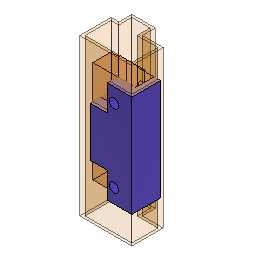
design (Autodesk Fusion 360 design; units mm, degrees)
Autodesk Fusion 360 part; units mm, degrees
note: some values were not read from the file. Chosen so that the rebuilt part matches the saved one: which bodies a step acts on.
sketch "Sketch1" plane through (0, 0, 0) normal (0, 0, 1) x (1, 0, 0) in component "铝槽"
  line L0 (0, 0) -> (18, 0)
  line L1 (18, 0) -> (18, 10)
  line L2 (18, 10) -> (10, 10)
  line L3 (10, 10) -> (10, 15)
  line L4 (10, 15) -> (3, 15)
  line L5 (3, 15) -> (3, 10)
  line L6 (3, 10) -> (0, 10)
  line L7 (0, 10) -> (0, 0)
  line L8 (-1, -1) -> (19, -1)
  line L9 (19, -1) -> (19, 11)
  line L10 (19, 11) -> (11, 11)
  line L11 (11, 11) -> (11, 16)
  line L12 (11, 16) -> (2, 16)
  line L13 (2, 16) -> (2, 11)
  line L14 (2, 11) -> (-1, 11)
  line L15 (-1, 11) -> (-1, -1)
  dimension "d1" = 18
  dimension "d2" = 10
  dimension "d3" = 8
  dimension "d4" = 5
  dimension "d5" = 7
  dimension "d6" = 1
  constraint coincident L0.start L7.end
  constraint horizontal L0
  constraint perpendicular L0 L1
  constraint perpendicular L1 L2
  constraint perpendicular L2 L3
  constraint perpendicular L3 L4
  constraint perpendicular L4 L5
  constraint perpendicular L5 L6
  constraint perpendicular L0 L7
  constraint equal L3 L5
  measures "d1" distance of L0.start L0.end
  measures "d2" distance of L0.end L1.end
  measures "d3" distance of L1.end L2.end
  measures "d4" distance of L2.end L3.end
  measures "d5" distance of L3.end L4.end
extrude "Extrude1" add sketch "Sketch1" along normal blind 60 makes body 1 in component "铝槽"
sketch "Sketch1 (2)" plane through (0, 0, 0) normal (0, 1, 0) x (1, 0, 0) in component "门铰"
  line L0 (0, -19.5) -> (0, 19.5)
  line L1 (-16, -9.5) -> (-16, 9.5)
  line L2 (0, -19.5) -> (-9.5, -19.5)
  line L3 (0, 19.5) -> (-9.5, 19.5)
  line L4 (-16, -9.5) -> (-9.5, -9.5)
  line L5 (-9.5, -9.5) -> (-9.5, -19.5)
  line L6 (-16, 9.5) -> (-9.5, 9.5)
  line L7 (-9.5, 9.5) -> (-9.5, 19.5)
  line L8 (0, 0) -> (-16, 0) construction
  circle A0 centre (-6.9, -14) radius 1.75
  circle A1 centre (-6.9, 14) radius 1.75
  dimension "d9" = 39
  dimension "d10" = 19
  dimension "d11" = 9.5
  dimension "d12" = 16
  dimension "d14" = 3.5
  dimension "d15" = 6.9
  dimension "d16" = 28
  constraint vertical L0
  constraint midpoint L8.start L0
  constraint vertical L1
  constraint perpendicular L0 L2
  constraint perpendicular L0 L3
  constraint equal L2 L3
  constraint perpendicular L1 L4
  constraint vertical L5
  constraint perpendicular L1 L6
  constraint vertical L7
  constraint equal L5 L7
  constraint coincident L8.start origin
  constraint midpoint L1 L8.end
  constraint symmetric L8 A0 A1
  measures "d9" distance of L0.start L0.end
  measures "d10" distance of L1.start L1.end
  measures "d11" distance of L0.start L2.end
  measures "d12" distance of L0 L1
  measures "d14" diameter of A0
  measures "d15" distance of L0 A0.centre
  measures "d16" distance of A0.centre A1.centre
extrude "Extrude1'" add sketch "Sketch1 (2)" along normal blind 11 separate body makes body 2 in component "门铰"
ref_plane "WorkPlane1" through (0, 5.5, 0) normal (1, 0, 0) x (0, 0, -1) in component "门铰"
sketch "Sketch2" plane through (0, 5.5, 0) normal (1, 0, 0) x (0, 1, 0) in component "门铰"
  line L0 (-5.5, 9.5) -> (-1.5, 9.5)
  line L1 (-5.5, -9.5) -> (-1.5, -9.5)
  line L2 (-5.5, 19.5) -> (-5.5, -19.5)
  line L3 (-5.5, -19.5) -> (5.5, -19.5)
  line L4 (5.5, -19.5) -> (5.5, 19.5)
  line L5 (5.5, 19.5) -> (-5.5, 19.5)
  line L6 (-1.5, 9.5) -> (-1.5, 19.5)
  line L7 (-1.5, -9.5) -> (-1.5, -19.5)
  line L8 (-1.5, 9.5) -> (5.5, 9.5)
  line L9 (-1.5, -9.5) -> (5.5, -9.5)
  point P0 (-5.5, 9.5)
  point P1 (-5.5, -9.5)
  dimension "d20" = 4
  constraint coincident P0 L0.start
  constraint horizontal L0
  constraint coincident P1 L1.start
  constraint horizontal L1
  constraint equal L0 L1
  constraint coincident L5 L6.end
  constraint perpendicular L5 L6
  constraint coincident L3 L7.end
  constraint perpendicular L3 L7
  constraint coincident L4 L8.end
  constraint perpendicular L4 L8
  constraint coincident L4 L9.end
  constraint perpendicular L4 L9
  measures "d20" distance of P0 L0.end
extrude "Extrude2" cut sketch "Sketch2" against normal up to surface (7 mm away) from surface at -2.5 contours L4 L5 L6 L8 | L3 L4 L7 L9 bodies 2 in component "门铰"
combine "Combine1" operation cut target body 1 tool bodies 2 body 2 seen with x (1, 0, 0) y (0, 1, 0) z (0, 0, 1) at (19, -1, 30) keep tools makes body 3 at (13.8413, -0.6667, 44.1742) makes body 4 at (13.8413, -0.6667, 16.1742) in component "铝槽"
sketch "Sketch1 (3)" plane through (0, 11.9627, 0) normal (0, 1, 0) x (-1, 0, 0) in component "填块"
  line L0 (-12.0433, -6.2222) -> (-3.0433, -6.2222)
  line L1 (-3.0433, -6.2222) -> (-3.0433, 53.7778)
  line L2 (-3.0433, 53.7778) -> (-12.0433, 53.7778)
  line L3 (-12.0433, 53.7778) -> (-12.0433, -6.2222)
  circle A0 centre (-13.1433, 37.7778) radius 1.75
  circle A1 centre (-13.1433, 9.7778) radius 1.75
  line L4 (-4.0433, 33.2778) -> (-17.5433, 33.2778)
  line L5 (-17.5433, 33.2778) -> (-17.5433, 43.2778)
  line L6 (-17.5433, 43.2778) -> (-20.0433, 43.2778)
  line L7 (-20.0433, 43.2778) -> (-20.0433, 4.2778)
  line L8 (-20.0433, 4.2778) -> (-17.5433, 4.2778)
  line L9 (-17.5433, 4.2778) -> (-17.5433, 14.2778)
  line L10 (-17.5433, 14.2778) -> (-4.0433, 14.2778)
  line L11 (-4.0433, 14.2778) -> (-4.0433, 33.2778)
  line L12 (-1.0433, -6.2222) -> (-1.0433, 53.7778)
  line L13 (-11.0433, -6.2222) -> (-11.0433, 53.7778)
  line L14 (-17.5433, 43.2778) -> (-1.0433, 43.2778)
  line L15 (-17.5433, 4.2778) -> (-1.0433, 4.2778)
  line L16 (-1.0433, 4.2778) -> (-1.0433, 43.2778)
  line L17 (-17.5433, 35.7778) -> (-7.5433, 35.7778)
  line L18 (-17.5433, 11.7778) -> (-7.5433, 11.7778)
  line L19 (-7.5433, 33.2778) -> (-7.5433, 43.2778)
  line L20 (-7.5433, 14.2778) -> (-7.5433, 4.2778)
  dimension "d36" = 2.5
  dimension "d37" = 2.5
  dimension "d38" = 3.5
  dimension "d39" = 3.5
  constraint coincident L5.end L6.start
  constraint coincident L12 L14.end
  constraint perpendicular L12 L14
  constraint coincident L8.end L9.start
  constraint coincident L12 L15.end
  constraint perpendicular L12 L15
  constraint coincident L5 L17.start
  constraint perpendicular L1 L17
  constraint coincident L9 L18.start
  constraint perpendicular L9 L18
  constraint coincident L14 L19.end
  constraint perpendicular L14 L19
  constraint coincident L15 L20.end
  constraint perpendicular L15 L20
  constraint coincident L4 L19.start
  constraint coincident L17.end L19
  constraint coincident L10 L20.start
  constraint coincident L18.end L20
  measures "d36" distance of L4 L17
  measures "d37" distance of L10 L18
  measures "d38" distance of L13 L19
  measures "d39" distance of L13 L20
extrude "Extrude1''" add sketch "Sketch1 (3)" along normal blind 1 separate body contours L3 A1 L9 L15 L18 | L3 A1 L13 L15 L18 | L13 L15 L18 L20 | L1 L4 L10 L11 L14 L15 L19 L20 | L1 L12 L14 L15 L16 | L13 L14 L17 L19 | L3 A0 L5 L14 L17 | L3 A0 L13 L14 L17 makes body 5 in component "填块"
extrude "Extrude2'" add 1 faces at (6.0433, 12.9627, 40.7778) along direction (0, 1, 0) up to surface (6 mm away) on bodies 5 bodies 5 in component "填块"
ref_plane "WorkPlane1" through (9.2933, 15.4627, 43.2778) normal (0, 0, 1) x (1, 0, 0) in component "填块"
sketch "Sketch3" plane through (9.2933, 15.4627, 43.2778) normal (0, 0, 1) x (1, 0, 0) in component "填块"
  line L0 (-5.25, 3.5) -> (-5.25, 8.5)
  line L1 (1.75, 8.5) -> (1.75, 3.5)
  line L2 (-5.25, 6.5) -> (1.75, 6.5)
  line L3 (8.25, 3.5) -> (-8.25, 3.5)
  dimension "d64" = 3
  constraint coincident L0 L2.start
  constraint coincident L1 L2.end
  constraint perpendicular L1 L2
  measures "d64" distance of L2 L3
extrude "Extrude5" add sketch "Sketch3" against normal up to surface (39 mm away) bodies 5 in component "填块"
chamfer "Chamfer1" distance 2.5 angle 45 2 edges at (7.5433, 21.9627, 43.2778) (7.5433, 21.9627, 4.2778) on bodies 5 in component "填块"
chamfer "Chamfer2" distance 7 distance2 3.5 2 edges at (7.5433, 18.9627, 13.0278) (7.5433, 18.9627, 34.5278) measured on face at (7.5433, 14.296, 12.6112) measured on face at (7.5433, 14.296, 34.1112) on bodies 5 in component "填块"
component "铝槽" placed x (1, 0, 0) y (0, 1, 0) z (0, 0, 1) at (-0.6055, -5.4112, -5.6974)
component "门铰" placed x (1, 0, 0) y (0, 1, 0) z (0, 0, 1) at (18.3945, -6.4112, 24.3026)
component "填块" placed x (1, 0, 0) y (0, 1, 0) z (0, 0, 1) at (-1.6488, -14.374, 0.5248)
hidden bodies 3 4
equation "d37 = ( d36 )"
equation "d39 = d38"
